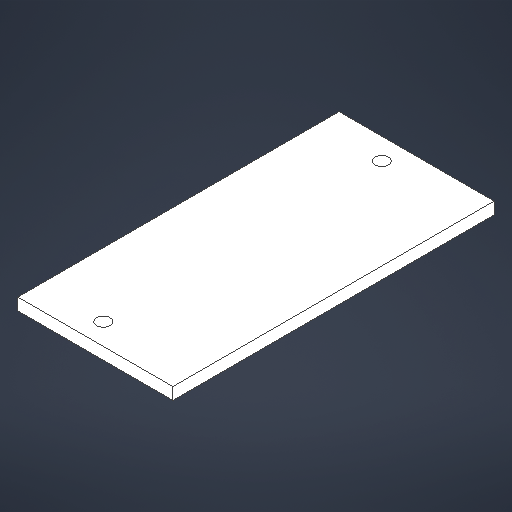
# Autodesk Inventor part: TapaBatería
Saved by Autodesk Inventor 2026.1 (Build 301233020, 233B)
## iProperties
Created: 2025-11-24
Part Number: TapaBatería
Material: Generic
Document SubType Name: Modeling
Designer: Tito Luyo Murata
Density: 1 g/cm^3
Appearance: Default
Author: Tito Luyo Murata
Autodesk Inventor part; units mm, degrees
ref_plane "YZ Plane" through (0, 0, 0) normal (1, 0, 0) x (0, 1, 0)
ref_plane "XZ Plane" through (0, 0, 0) normal (0, 1, 0) x (-1, 0, 0)
ref_plane "XY Plane" through (0, 0, 0) normal (0, 0, 1) x (1, 0, 0)
sketch "Sketch1" plane through (0, 0, 0) normal (0, 1, 0) x (-1, 0, 0)
  line L0 (0, -0.2057) -> (36.2, -0.2057)
  line L1 (36.2, -0.2057) -> (36.2, -75.2057)
  line L2 (36.2, -75.2057) -> (0, -75.2057)
  line L3 (0, -75.2057) -> (0, -0.2057)
  circle A0 centre (21.24, -5.2057) radius 1.6
  circle A1 centre (21.24, -70.2057) radius 1.6
  point P0 (0, 0)
  dimension "d0" = 36.2
  dimension "d1" = 75
  dimension "d2" = 3.2
  dimension "d3" = 14.96
  dimension "d4" = 5
  dimension "d5" = 3.2
  dimension "d6" = 14.96
  dimension "d7" = 5
  constraints: 8 end point, 2 centre point, 2 parallel, 1 horizontal, 1 perpendicular
  measures "d0" distance of L1.end L2.end
  measures "d1" distance of L0.end L1.end
  measures "d2" diameter of A0
  measures "d3" distance from line of A0.centre L1
  measures "d4" distance from line of A0.centre L0
  measures "d5" diameter of A1
  measures "d6" distance from line of A1.centre L1
  measures "d7" distance from line of L2 A1.centre
extrude "Extrusion1" add sketch "Sketch1" along normal blind 2.8
body "Solid1"
